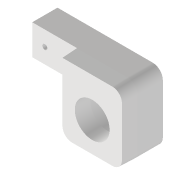
# Autodesk Inventor part: IM_Lensholder_motorized_lensadapter
Saved by Autodesk Inventor 2022 (Build 260153000, 153)
## iProperties
Created: 2023-08-15
Part Number: IM_Lensholder_motorized_lensadapter
Material: Generisch
Document SubType Name: Modeling
Designer: diederichbenedict
Density: 1 g/cm^3
Appearance: Vorgabe
Author: diederichbenedict
Autodesk Inventor part; units mm, degrees
ref_plane "YZ Plane" through (0, 0, 0) normal (1, 0, 0) x (0, 1, 0)
ref_plane "XZ Plane" through (0, 0, 0) normal (0, 1, 0) x (-1, 0, 0)
ref_plane "XY Plane" through (0, 0, 0) normal (0, 0, 1) x (1, 0, 0)
sketch "Skizze1" plane through (0, 0, 0) normal (0, 0, 1) x (1, 0, 0)
  circle A0 centre (2.5, -3) radius 0.5 projected
  line L0 (0, 0) -> (0, -6) projected
  line L1 (0, -6) -> (5, -6) projected
  line L2 (5, 0) -> (5, -6) projected
  line L3 (0, 0) -> (5, 0) projected
  circle A1 centre (14.8779, -7.8108) radius 3.9802 projected
  line L4 (5, 0) -> (18.8779, 0)
  line L5 (20.8779, -2) -> (20.8779, -11.8108)
  line L6 (18.8779, -13.8108) -> (11.8779, -13.8108)
  line L7 (9.8779, -11.8108) -> (9.8779, -6)
  line L8 (9.8779, -6) -> (5, -6)
  arc A2 (9.8779, -11.8108) -> (11.8779, -13.8108) centre (11.8779, -11.8108) ccw
  arc A3 (18.8779, -13.8108) -> (20.8779, -11.8108) centre (18.8779, -11.8108) ccw
  arc A4 (20.8779, -2) -> (18.8779, 0) centre (18.8779, -2) ccw
  line L9 (0, -4.579) -> (9.9072, -4.579)
  line L10 (9.9072, -4.579) -> (9.9072, -13.8108)
  line L11 (9.9072, -13.8108) -> (11.8779, -13.8108)
  circle A5 centre (2.5, -3) radius 1
  circle A6 centre (14.8779, -7.8108) radius 3.35
  point P0 (9.9072, -12.1516)
  dimension "d0" = 6
  dimension "d1" = 5
  dimension "d2" = 6
  dimension "d3" = 2
  dimension "d9" = 2
  dimension "d10" = 6.7
  constraints: 16 end point, 6 point on circle, 6 tangent, 5 centre point, 5 perpendicular, 2 coincident, 2 equal radius, 2 horizontal, 1 collinear, 1 point on line
  measures "d0" distance from line of L5 A1.centre
  measures "d1" distance from line of A1.centre L7
  measures "d2" distance from line of L6 A1.centre
  measures "d3" radius of A2
  measures "d9" diameter of A5
  measures "d10" diameter of A6
extrude "Extrusion1" add sketch "Skizze1" along normal blind 5 contours L3 L2 L9 L0 | L4 A4 L5 A3 L6 A2 L10 L9 L2 | A1
